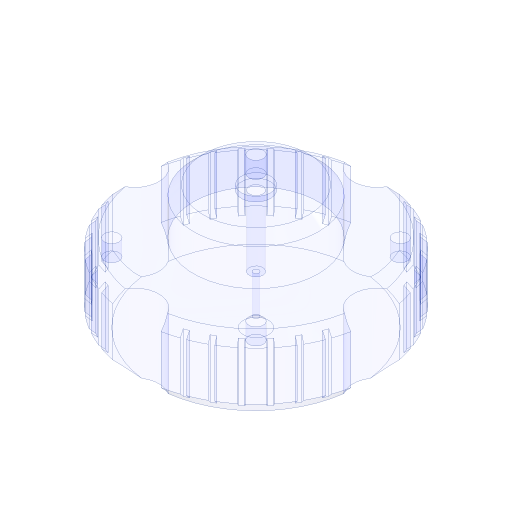
# Autodesk Inventor part: cpd_lowrcf_1.3_p1_20230620
Saved by Autodesk Inventor 2024 (Build 280153000, 153)
## iProperties
Created: 2021-12-07
Part Number: cpd_lowrcf_1.3_p1_20230620
Material: Generic
Document SubType Name: Modeling
Designer: tomos
Density: 1 g/cm^3
Appearance: Clear - Blue
Author: tomos
Autodesk Inventor part; units mm, degrees
ref_plane "YZ Plane" through (0, 0, 0) normal (1, 0, 0) x (0, 1, 0)
ref_plane "XZ Plane" through (0, 0, 0) normal (0, 1, 0) x (-1, 0, 0)
ref_plane "XY Plane" through (0, 0, 0) normal (0, 0, 1) x (1, 0, 0)
sketch "Sketch1" plane through (0, 0, 0) normal (0, 0, 1) x (1, 0, 0)
  line L0 (0, 0) -> (0, 7.0545) construction
  line L1 (0, 0) -> (4.1333, 0) construction
  line L2 (0.7, 0) -> (0.7, 4.75)
  line L3 (12.5, -8) -> (0.3, -8)
  line L4 (0.3, 0) -> (0.7, 0)
  line L5 (6.425, 4.75) -> (6.425, 0)
  line L6 (6.425, 0) -> (12.5, 0)
  line L7 (12.5, 0) -> (12.5, -8)
  line L8 (0.7, 4.75) -> (6.425, 4.75)
  line L9 (0.3, -8) -> (0.3, -3)
  line L10 (0.3, -3) -> (0.7, -3)
  line L11 (0.7, -3) -> (0.7, 0)
  dimension "d0" = 0.7
  dimension "d8" = 8
  dimension "d9" = 6.425
  dimension "d10" = 12.5
  dimension "d66" = 4.75
  dimension "d67" = 4.75
  dimension "d71" = 0.3
  dimension "d72" = 5
  constraints: 24 end point, 5 perpendicular, 3 vertical, 2 horizontal, 2 point on line, 1 collinear
  measures "d0" distance between parallel lines of L2 L0
  measures "d8" distance between parallel lines of L3 L1
  measures "d9" distance between parallel lines of L5 L0
  measures "d10" distance between parallel lines of L7 L0
  measures "d66" distance between parallel lines of L1 L8
  measures "d67" distance between parallel lines of L6 L8
  measures "d71" distance between parallel lines of L0 L9
  measures "d72" distance from line of L3.end L10
revolve "Revolution1" add sketch "Sketch1" angle 360 about axis through (0, 0, 0) along (0, 1, 0)
chamfer "Chamfer2" [suppressed]
chamfer "Chamfer3" distance 1 angle 45 1 edges at (-0.3, -8, 0)
sketch "Sketch5" plane through (0, -8, 0) normal (0, -1, 0) x (1, 0, 0)
  circle A0 centre (0, 0) radius 12.5
  circle A1 centre (0, 0) radius 12
  line L0 (0, 0) -> (-3.6414, 0) construction
  line L1 (-11.9974, 0.25) -> (-12.4975, 0.25)
  line L2 (-11.9974, -0.25) -> (-12.4975, -0.25)
  point P0 (-12.4975, -0.25)
  point P1 (-12.2474, -0.25)
  dimension "d34" = 25
  dimension "d35" = 24
  dimension "d33" = 0.25
  constraints: 6 end point, 4 coincident, 2 horizontal, 2 symmetric about line, 6 other
  measures "d33" distance between parallel lines of L1 L0
extrude "Extrusion2" [suppressed]
pattern_circular "Circular Pattern2" [suppressed]
sketch "Sketch6" plane through (0, 0, 0) normal (0, 1, 0) x (1, 0, 0)
  circle A0 centre (0, 0) radius 12.5
  circle A1 centre (0, 0) radius 0.7 construction
  line L0 (0, 0) -> (0, 16.4064) construction
  circle A2 centre (0, 12.5) radius 2.5
  point P0 (-2.4875, 12.25)
  point P1 (2.4875, 12.25)
  dimension "d41" = 25
  dimension "d42" = 5
  constraints: 2 end point, 1 centre point, 1 coincident, 1 point on line, 1 vertical, 3 other
  measures "d42" diameter of A2
extrude "Extrusion3" [suppressed]
pattern_circular "Circular Pattern3" [suppressed]
sketch "Sketch7" plane through (0, 0, -12.5) normal (0, 1, 0) x (1, 0, 0)
  circle A0 centre (0, -12.5) radius 0.7 construction
  circle A1 centre (0, -12.5) radius 10.5 construction
  line L0 (0, -12.5) -> (-15.963, -12.5) construction
  line L1 (0, -12.5) -> (-12.3969, -0.1031) construction
  circle A2 centre (-7.4246, -5.0754) radius 0.8
  dimension "d48" = 21
  dimension "d49" = 45
  dimension "d50" = 1.6
  constraints: 4 end point, 1 centre point, 1 coincident, 1 horizontal, 1 point on line, 3 other
  measures "d49" angle of L1 L0
  measures "d50" diameter of A2
extrude "Extrusion4" [suppressed]
chamfer "Chamfer4" [suppressed]
pattern_circular "Circular Pattern4" [suppressed]
sketch "Sketch8" plane through (0, 4.75, 0) normal (0, 1, 0) x (1, 0, 0)
  line L0 (-11.2038, 0) -> (0, 0) construction
  line L1 (0, 0) -> (0, 15.4085) construction
  circle A0 centre (0, 0) radius 0.7 projected
  circle A1 centre (0, 0) radius 1.5
  dimension "d68" = 3
  constraints: 4 end point, 1 centre point, 1 coincident, 1 horizontal, 1 perpendicular
  measures "d68" diameter of A1
extrude "Extrusion5" [suppressed]
chamfer "Chamfer6" distance 2 angle 45 1 edges at (-12.5, -8, 0)
chamfer "Chamfer7" distance 1 angle 45 2 edges at (-12.5, 0, 0) (-6.425, 4.75, 0)
sketch "Sketch9" plane through (0, -8, 0) normal (0, -1, 0) x (1, 0, 0)
  circle A0 centre (0, 0) radius 12.5 construction
  circle A1 centre (0, 0) radius 0.7 construction
  circle A2 centre (0, 0) radius 12 construction
  line L0 (0, 0) -> (0, 22.0081) construction
  line L1 (0, 0) -> (34.9599, 0) construction
  circle A3 centre (0, 0) radius 12.5 projected
  circle A4 centre (0, 0) radius 12
  circle A5 centre (0, 0) radius 1.3 projected
  circle A6 centre (0, 0) radius 12
  circle A7 centre (0, 0) radius 12.5
  line L2 (0.25, 12.4975) -> (0.25, 11.9974)
  line L3 (-0.25, 12.4975) -> (-0.25, 11.9974)
  dimension "d83" = 24
  dimension "d84" = 25
  dimension "d79" = 25
  dimension "d80" = 24
  dimension "d85" = 0.25
  constraints: 8 end point, 5 coincident, 3 centre point, 2 symmetric about line, 2 vertical, 1 concentric, 1 horizontal, 6 other
  measures "d79" diameter of A0
  measures "d80" diameter of A2
  measures "d85" distance between parallel lines of L0 L2
extrude "Extrusion6" cut sketch "Sketch9" against normal blind 12.75 contours L2 A4 L3 A3 picked at (-0.1944, 12.1649)
pattern_circular "Circular Pattern5" count 36 over 360 about axis through (0, 0.875, 0) along (0, -1, 0) of "Extrusion6"
sketch "Sketch10" plane through (0, -8, 0) normal (0, -1, 0) x (1, 0, 0)
  circle A0 centre (0, 0) radius 12.5 construction
  line L0 (0, 0) -> (0, 20.459) construction
  line L1 (0, 0) -> (24.7433, 0) construction
  circle A1 centre (12.5, 0) radius 2.5
  dimension "d91" = 25
  dimension "d92" = 5
  constraints: 4 end point, 2 coincident, 1 centre point, 1 horizontal, 1 horizontal alignment, 1 point on line, 1 vertical, 2 other
  measures "d92" diameter of A1
extrude "Extrusion7" cut sketch "Sketch10" against normal blind 8
pattern_circular "Circular Pattern6" count 4 over 360 about axis through (0, 0.875, 0) along (0, -1, 0) of "Extrusion7"
sketch "Sketch11" plane through (0, 4.75, 0) normal (0, 1, 0) x (1, 0, 0)
  line L0 (0, 0) -> (0, 19.5723) construction
  line L1 (0, 0) -> (39.8368, 0) construction
  circle A0 centre (0, 0) radius 12.5 construction
  circle A1 centre (0, 0) radius 1.5
  dimension "d98" = 25
  dimension "d99" = 3
  constraints: 4 end point, 2 centre point, 2 coincident, 1 horizontal, 1 vertical
  measures "d98" diameter of A0
  measures "d99" diameter of A1
extrude "Extrusion8" cut sketch "Sketch11" against normal blind 0.5
sketch "Sketch12" plane through (12.5, 0, 0) normal (0, 1, 0) x (1, 0, 0)
  circle A0 centre (-12.5, 0) radius 10.5 construction
  line L0 (-12.5, 0) -> (-33.0857, 0) construction
  line L1 (-12.5, 0) -> (-26.7842, -14.2842) construction
  circle A1 centre (-19.9246, -7.4246) radius 0.75
  dimension "d102" = 21
  dimension "d103" = 45
  dimension "d104" = 1.5
  constraints: 4 end point, 2 coincident, 1 centre point, 1 horizontal, 1 point on line, 3 other
  measures "d103" angle of L0 L1
  measures "d104" diameter of A1
extrude "Extrusion9" cut sketch "Sketch12" against normal blind 1.7
pattern_circular "Circular Pattern7" count 4 over 360 about axis through (0, 4.75, 0) along (0, -1, 0) of "Extrusion9"
equation "\"rotor_diameter\" = 0.7"
equation "\"tolerancefactor\" = 1.1"
equation "\"rotor_length\" = 4.65"
equation "\"cutpipette_enddiameter\" = 1.181"
body "Solid1"
